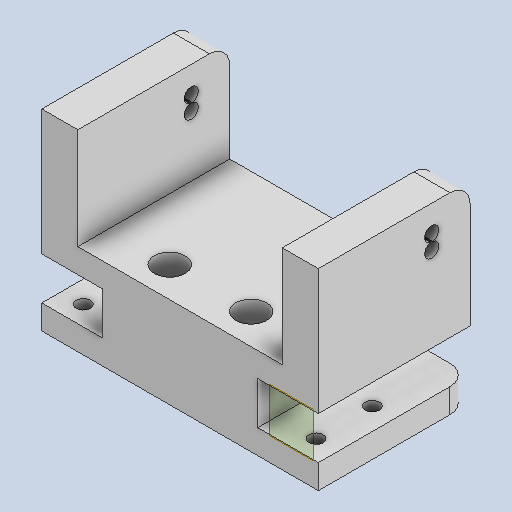
# Autodesk Inventor part: 30_Cube_Z_Focus_Drylin_manual_base_lightsheet_v3
Saved by Autodesk Inventor 2022 (Build 260153000, 153)
## iProperties
Created: 2021-11-07
Part Number: 30_Cube_Z_Focus_Drylin_manual_base_lightsheet_v3
Material: Generic
Document SubType Name: Modeling
Designer: diederichbenedict
Density: 1 g/cm^3
Appearance: Default
Author: diederichbenedict
Autodesk Inventor part; units mm, degrees
ref_plane "YZ Plane" through (0, 0, 0) normal (1, 0, 0) x (0, 1, 0)
ref_plane "XZ Plane" through (0, 0, 0) normal (0, 1, 0) x (-1, 0, 0)
ref_plane "XY Plane" through (0, 0, 0) normal (0, 0, 1) x (1, 0, 0)
ref_plane "Work Plane1" through (-1.4137, -31.0503, -3.3468) normal (0, 0, -1) x (-1, 0, 0)
sketch "Sketch1" plane through (-1.4137, -31.0503, -3.3468) normal (0, 0, -1) x (-1, 0, 0)
  line L0 (41.325, -8) -> (41.325, 0)
  line L1 (29.55, -8) -> (29.55, 0)
  line L2 (44, -8) -> (44, 0) projected
  line L3 (14, 34) -> (14, 6)
  line L4 (14, 5) -> (29.35, 5)
  line L5 (29.35, 5) -> (29.35, -13)
  line L6 (29.35, -13) -> (14, -13)
  line L7 (14, -13) -> (14, 5)
  line L8 (29.35, 5) -> (41.325, 5)
  line L9 (41.325, 5) -> (41.325, 0.2)
  line L10 (41.325, 0.2) -> (29.35, 0.2)
  line L11 (29.35, 0.2) -> (29.35, 5)
  line L12 (29.35, -13) -> (41.325, -13)
  line L13 (41.325, -13) -> (41.325, -8.2)
  line L14 (41.325, -8.2) -> (29.35, -8.2)
  line L15 (29.35, -8.2) -> (29.35, -13)
  line L16 (30, 0) -> (34, 0) projected
  line L17 (34, -8) -> (30, -8) projected
  line L18 (41.325, 5) -> (34.2, 5)
  line L19 (34.2, 5) -> (34.2, 25)
  line L20 (34.2, 25) -> (41.325, 25)
  line L21 (41.325, 25) -> (41.325, 5)
  point P0 (-1.4137, 31.0503)
  point P1 (34, 21.1361)
  point P2 (34.2, 5)
  point P3 (29.35, -8.2)
  point P4 (29.35, 0.2)
  dimension "d0" = 5
  dimension "d1" = 0
  dimension "d2" = 0.2
  dimension "d3" = 5
  dimension "d4" = 0.2
  dimension "d5" = 0.2
  dimension "d6" = 20
  dimension "d7" = 0.2
  constraints: 38 end point, 8 parallel, 4 horizontal, 4 perpendicular, 3 vertical, 1 point on line, 7 other
  measures "d0" distance from line of L1.end L4
  measures "d1" distance between parallel lines of L3 L7
  measures "d2" distance between parallel lines of L5 L1
  measures "d3" vertical distance of L1.start L5.end
  measures "d4" distance between parallel lines of L16 L10
  measures "d5" distance between parallel lines of L14 L17
  measures "d6" distance of L18.end L19.end
  measures "d7" distance from line of point (34, 21.136) L19
extrude "Extrusion1" add sketch "Sketch1" along normal blind 30
sketch "Sketch2" plane through (-35.6137, -26.0503, -3.3468) normal (0, 1, 0) x (1, 0, 0)
  circle A0 centre (12.1511, -14.3969) radius 3 construction
  circle A1 centre (12.1511, 6) radius 3.05
  line L0 (-7.125, 0) -> (0, 0) projected
  point P0 (35.6137, -3.3468)
  dimension "d10" = 6.1
  dimension "d13" = 6
  constraints: 1 centre point
  measures "d10" diameter of A1
  measures "d13" distance from line of A1.centre L0
extrude "Extrusion2" cut sketch "Sketch2" against normal blind 25.4
sketch "Sketch3" plane through (-42.7387, -30.8503, -3.3468) normal (-1, 0, 0) x (0, 0, 1)
  circle A0 centre (-22.3882, 16.8) radius 1.4 projected
  point P0 (3.3468, 30.8503)
extrude "Extrusion3" cut sketch "Sketch3" against normal blind 30
fillet "Fillet1" radius 4 2 edges at (-39.1762, -6.0503, -33.3468) (-42.7387, -41.6503, -33.3468)
mirror "Mirror1" about plane through (-15.4137, -26.0503, -3.3468) normal (1, 0, 0) of "Extrusion1", "Extrusion2", "Extrusion3", "Fillet1"
sketch "Sketch4" plane through (-42.7387, -44.0503, -29.3468) normal (0, -1, 0) x (1, 0, 0)
  arc A0 (50.65, -4) -> (54.65, 0) centre (50.65, 0) ccw projected
  line L0 (54.65, 26) -> (54.65, 0) projected
  line L1 (0, 26) -> (54.65, 26) projected
  line L2 (0, 26) -> (0, 0) projected
  arc A1 (0, 0) -> (4, -4) centre (4, 0) ccw projected
  line L3 (4, -4) -> (50.65, -4) projected
  circle A2 centre (35.3739, 20) radius 3.05 projected
  circle A3 centre (19.2761, 20) radius 3.05 projected
  circle A4 centre (4.325, 31.6031) radius 1.45 projected
  circle A5 centre (4.325, 22.1383) radius 1.4
  circle A6 centre (4.325, 10.7325) radius 1.4
  circle A7 centre (50.325, 22.1383) radius 1.4
  circle A8 centre (50.325, 11) radius 1.4
  point P0 (42.7387, 29.3468)
  dimension "d17" = 2.8
  dimension "d18" = 2.8
  dimension "d19" = 2.8
  dimension "d20" = 2.8
  dimension "d21" = 4.325
  dimension "d22" = 4.325
  dimension "d23" = 4.325
  constraints: 4 centre point
  measures "d17" diameter of A5
  measures "d18" diameter of A6
  measures "d19" diameter of A7
  measures "d20" diameter of A8
  measures "d21" distance from line of A5.centre L2
  measures "d22" distance from line of A7.centre L0
  measures "d23" distance from line of A8.centre L0
extrude "Extrusion4" cut sketch "Sketch4" against normal blind 30 contours A5 | A6 | A7 | A8
sketch "Skizze5" plane through (11.9113, -30.8503, -3.3468) normal (1, 0, 0) x (0, 0, -1)
  circle A0 centre (22.3882, 19.5744) radius 1.4 projected
  circle A1 centre (22.3882, 19.5744) radius 1.4
  point P0 (-3.3468, 30.8503)
  dimension "d26" = 2.8
  constraints: 1 centre point, 1 coincident
  measures "d26" diameter of A1
extrude "Extrusion5" cut sketch "Skizze5" against normal through all
equation "\"d22\" = d21"
equation "\"d23\" = d21"
body "Solid1"
